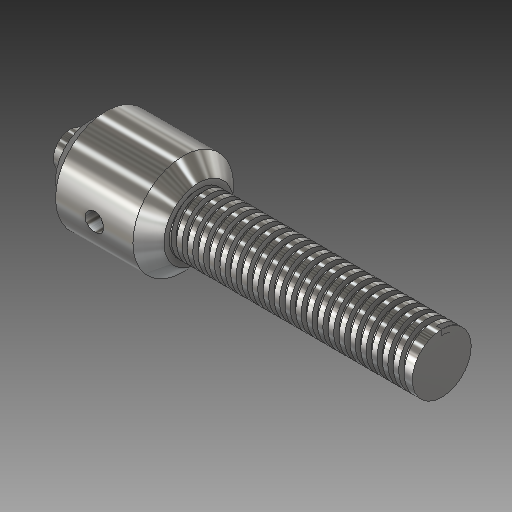
# Autodesk Inventor part: Screw Spindle
Saved by Autodesk Inventor 2018 (Build 220112000, 112)
## iProperties
Created: 2019-08-31
Part Number: Screw Spindle
Material: Generic
Document SubType Name: Modeling
Designer: HP
Density: 1 g/cm^3
Appearance: Chrome - Polished
Author: HP
Autodesk Inventor part; units mm, degrees
ref_plane "YZ Plane" through (0, 0, 0) normal (1, 0, 0) x (0, 1, 0)
ref_plane "XZ Plane" through (0, 0, 0) normal (0, 1, 0) x (-1, 0, 0)
ref_plane "XY Plane" through (0, 0, 0) normal (0, 0, 1) x (1, 0, 0)
sketch "Sketch1" plane through (0, 0, 0) normal (0, 0, 1) x (1, 0, 0)
  line L0 (0, 0) -> (0, 11)
  line L1 (0, 11) -> (13, 11)
  line L2 (0, 0) -> (240, 0)
  line L3 (240, 0) -> (240, 19)
  line L4 (240, 19) -> (83, 19)
  line L5 (13, 11) -> (13, 22.5)
  line L6 (23, 32.5) -> (73, 32.5)
  line L7 (83, 22.5) -> (73, 32.5)
  line L8 (83, 22.5) -> (83, 19)
  line L9 (23, 32.5) -> (13, 22.5)
  dimension "d0" = 11
  dimension "d3" = 19
  dimension "d5" = 11.5
  constraints: 20 end point, 3 perpendicular, 3 vertical, 1 horizontal
  measures "d0" distance of L0.start L0.end
  measures "d3" distance of L2.end L3.end
  measures "d5" distance of L1.end L5.end
revolve "Revolution1" add sketch "Sketch1" angle 360 about axis through (0, 0, 0) along (1, 0, 0)
sketch "Sketch2" plane through (0, 0, 0) normal (0, 0, 1) x (1, 0, 0)
  line L0 (240, -19) -> (240, 19) projected
  line L1 (240, 19) -> (236.5, 19)
  line L2 (83, 19) -> (240, 19) projected
  line L3 (236.5, 19) -> (236.5, 15.5)
  line L4 (236.5, 15.5) -> (240, 15.5)
  line L5 (240, 15.5) -> (240, 19)
  point P0 (0, 0)
  constraints: 8 end point, 2 point on line, 1 collinear, 1 vertical
coil "Coil1" sketch "Sketch2" operation cut axis through (-10, 0, 0) along (-1, 0, 0) pitch 7 turns 22.285714 hand right
sketch "Sketch3" plane through (0, 0, 0) normal (0, 0, 1) x (1, 0, 0)
  circle A0 centre (48, -0.9408) radius 6
  point P0 (0, 0)
  dimension "d22" = 12
  constraints: 1 centre point
  measures "d22" diameter of A0
extrude "Extrusion1" cut sketch "Sketch3" along normal through all both and the other way through all
sketch "Sketch4" plane through (0, 0, 0) normal (-1, 0, 0) x (0, 0, 1)
  circle A0 centre (0, 0) radius 6
  dimension "d25" = 12
  constraints: 1 centre point, 1 coincident
  measures "d25" diameter of A0
extrude "Extrusion2" cut sketch "Sketch4" against normal blind 35
thread "Thread1" size "M12x1.75" class "6H" standard "ANSI Metric M Profile" length 30 offset 5
body "Solid1"
